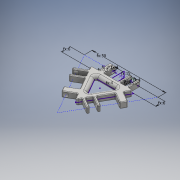
# Autodesk Inventor part: triangle
Saved by Autodesk Inventor 2016 (Build 200138000, 138)
## iProperties
Created: 2016-11-12
Part Number: triangle
Material: Generic
Document SubType Name: Modeling
Designer: Chris
Density: 1 g/cm^3
Appearance: Default
Author: Chris
Autodesk Inventor part; units mm, degrees
ref_plane "XZ Plane" through (0, 0, 0) normal (0, 1, 0) x (-1, 0, 0)
ref_plane "XY Plane" through (0, 0, 0) normal (0, 0, 1) x (1, 0, 0)
sketch "Sketch1" plane through (0, 0, 0) normal (0, 0, 1) x (1, 0, 0)
  line L0 (25, 14.4338) -> (0, -28.8675) construction
  line L1 (0, -28.8675) -> (-25, 14.4338) construction
  line L2 (-25, 14.4338) -> (25, 14.4338) construction
  line L3 (14.6077, 8.4338) -> (0, -16.8675)
  line L4 (0, -16.8675) -> (-14.6077, 8.4338)
  line L5 (-14.6077, 8.4338) -> (14.6077, 8.4338)
  line L6 (-7.5, 14.4338) -> (7.5, 14.4338) construction
  line L7 (5.5, 14.4338) -> (9.5, 14.4338) construction
  line L8 (-9.5, 14.4338) -> (-5.5, 14.4338) construction
  line L9 (7.6795, 4.4338) -> (0, -8.8675)
  line L10 (0, -8.8675) -> (-7.6795, 4.4338)
  line L11 (-7.6795, 4.4338) -> (7.6795, 4.4338)
  point P0 (0, 0)
  point P1 (0, 0)
  point P2 (0, 14.4338)
  dimension "d0" = 50
  dimension "d2" = 15
  dimension "d4" = 4
  dimension "d5" = 6
  dimension "d6" = 4
  dimension "d7" = 4
  dimension "d18" = 6
  constraints: 24 end point, 7 coincident, 4 horizontal, 4 midpoint, 1 collinear, 11 other
  measures "d0" distance of L1.end L0.start
  measures "d2" distance of L6.start L6.end
  measures "d4" distance of L7.start L7.end
  measures "d5" distance between parallel lines of L5 L7
  measures "d6" distance of L8.start L8.end
  measures "d7" distance between parallel lines of L5 L11
  measures "d18" distance between parallel lines of L5 L2
extrude "Extrusion1" add sketch "Sketch1" along normal mid plane 4
sketch "Sketch2" plane through (0, 0, 0) normal (1, 0, 0) x (0, 1, 0)
  line L0 (8.4338, 2) -> (8.4338, -2) construction
  line L1 (8.4338, -2) -> (8.4338, 2) construction
  line L2 (8.4338, 2) -> (13.4338, 2) construction
  line L3 (12.4338, -2) -> (8.4338, -2) construction
  line L4 (8.4338, -2) -> (8.4338, 2) construction
  arc A0 (14.4338, -2) -> (14.4338, 2) centre (14.4338, 0) ccw
  line L5 (14.4338, -2) -> (8.4338, -2)
  line L6 (8.4338, -2) -> (8.4338, 2)
  line L7 (8.4338, 2) -> (14.4338, 2)
  line L8 (14.4338, -2) -> (16.4338, -2)
  line L9 (16.4338, -2) -> (16.4338, 2)
  line L10 (16.4338, 2) -> (14.4338, 2)
  point P0 (0, 0)
  point P1 (14.4338, 0)
  point P2 (14.4338, 0)
  constraints: 18 end point, 5 perpendicular, 3 horizontal, 3 tangent, 2 coincident, 2 point on circle, 2 point on line, 1 centre point, 1 parallel
ref_plane "Work Plane1" through (-9.5, 14.4338, 0) normal (1, 0, 0) x (0, 1, 0)
ref_plane "Work Plane2" through (-5.5, 14.4338, 0) normal (1, 0, 0) x (0, 1, 0)
ref_plane "Work Plane3" through (5.5, 14.4338, 0) normal (1, 0, 0) x (0, 1, 0)
ref_plane "Work Plane4" through (9.5, 14.4338, 0) normal (1, 0, 0) x (0, 1, 0)
extrude "Extrusion2" add sketch "Sketch2" along normal up to surface (4 mm away) from surface at -9.5
ref_plane "Work Plane5" through (4, 14.4338, 0) normal (1, 0, 0) x (0, 1, 0)
ref_plane "Work Plane6" through (11, 14.4338, 0) normal (1, 0, 0) x (0, 1, 0)
extrude "Extrusion3" add sketch "Sketch2" along normal up to surface (1.5 mm away) from surface at 4
extrude "Extrusion4" add sketch "Sketch2" along normal up to surface (1.5 mm away) from surface at 9.5
sketch "Sketch3" plane through (0, 0, 0) normal (0, 0, 1) x (1, 0, 0)
  line L0 (-9.5, 15.9338) -> (-9.5, 14.4338)
  line L1 (-5.5, 15.9338) -> (-5.5, 14.4338)
  line L2 (5.5, 15.9338) -> (5.5, 14.4338)
  line L3 (9.5, 15.9338) -> (9.5, 14.4338)
  line L4 (5.5, 14.4338) -> (9.5, 14.4338) construction
  line L5 (-7.5, 14.4338) -> (7.5, 14.4338) construction
  arc A0 (6, 14.4338) -> (5.5, 15.9338) centre (3.5, 14.4338) ccw
  arc A1 (9.5, 15.9338) -> (9, 14.4338) centre (11.5, 14.4338) ccw
  arc A2 (-9, 14.4338) -> (-9.5, 15.9338) centre (-11.5, 14.4338) ccw
  arc A3 (-5.5, 15.9338) -> (-6, 14.4338) centre (-3.5, 14.4338) ccw
  line L6 (9, 14.4338) -> (9.5, 14.4338)
  line L7 (6, 14.4338) -> (5.5, 14.4338)
  line L8 (-5.5, 14.4338) -> (-6, 14.4338)
  line L9 (-9, 14.4338) -> (-9.5, 14.4338)
  point P0 (0, 0)
  point P1 (5.475, 16.4338)
  dimension "d31" = 0.5
  dimension "d32" = 3
  dimension "d33" = 0.5
  constraints: 16 end point, 8 point on circle, 5 collinear, 5 point on line, 4 centre point, 4 coincident, 4 vertical, 3 equal radius, 2 horizontal alignment
  measures "d31" distance of L2.end L7.start
  measures "d32" diameter of point (-9.5, 15.934) L9
  measures "d33" distance of L9.start L0.end
revolve "Revolution1" cut sketch "Sketch3" angle 360 about axis through (-9, 14.4338, 0) along (-1, 0, 0) contours A2 L9 L0 | L1 L8 A3
revolve "Revolution2" add sketch "Sketch3" angle 360 about axis through (6, 14.4338, 0) along (-1, 0, 0) contours A0 L7 L2 | L3 L6 A1
pattern_circular "Circular Pattern1" count 3 over 360 about axis through (0, 0, -10) along (0, 0, 1) of "Extrusion4", "Extrusion3", "Extrusion2", "Revolution1", "Revolution2"
fillet "Fillet2" radius 1 6 edges at (14.6077, 8.4338, 0) (-14.6077, 8.4338, 0) (0, -16.8675, 0) (7.6795, 4.4338, 0) (-7.6795, 4.4338, 0) (0, -8.8675, 0)
fillet "Fillet3" radius 0.5 36 edges at (2.5538, -12.4441, 0) (4.5538, -8.98, 0) (5.3038, -7.681, 0) (10.0538, 0.5463, 0) (12.0538, 4.0104, 0) (9.5, 8.4338, 0) (5.5, 8.4338, 0) (4, 8.4338, 0) (-5.5, 8.4338, 0) (-9.5, 8.4338, 0) (-12.0538, 4.0104, 0) (-10.0538, 0.5463, 0) (-9.3038, -0.7528, 0) (-4.5538, -8.98, 0) (-2.5538, -12.4441, 0) (-12.8038, 5.3094, 0) (11, 8.4338, 0) (1.8038, -13.7432, 0) (8.7321, -17.7432, 0) (9.4821, -16.4441, 0) (11.4821, -12.98, 0) (12.2321, -11.681, 0) (16.9821, -3.4537, 0) (18.9821, 0.0104, 0) (11, 16.4338, 0) (9.5, 16.4338, 0) (5.5, 16.4338, 0) (4, 16.4338, 0) (-5.5, 16.4338, 0) (-9.5, 16.4338, 0) (-19.7321, 1.3094, 0) (-18.9821, 0.0104, 0) (-16.9821, -3.4537, 0) (-16.2321, -4.7528, 0) (-11.4821, -12.98, 0) (-9.4821, -16.4441, 0)
fillet "Fillet4" radius 2 12 edges at (3.8397, -2.2169, -2) (0, -7.8675, -2) (-3.8397, -2.2169, -2) (-6.8135, 3.9338, -2) (0, 4.4338, -2) (6.8135, 3.9338, -2) (0, 4.4338, 2) (-6.8135, 3.9338, 2) (-3.8397, -2.2169, 2) (0, -7.8675, 2) (3.8397, -2.2169, 2) (6.8135, 3.9338, 2)
chamfer "Chamfer1" distance 0.4 angle 45 144 edges at (13.0227, 5.6885, 2) (13.7417, 7.9338, 2) (12.1878, 8.4338, 2) (11.1464, 8.5802, 2) (11, 12.4338, 2) (10.8536, 16.2873, 2) (9.6464, 16.2873, 2) (9.5, 12.4338, 2) (9.3536, 8.5802, 2) (7.5, 8.4338, 2) (5.6464, 8.5802, 2) (5.5, 12.4338, 2) (5.3536, 16.2873, 2) (4.1464, 16.2873, 2) (4, 12.4338, 2) (3.8536, 8.5802, 2) (-0.75, 8.4338, 2) (-5.3536, 8.5802, 2) (-5.5, 12.4338, 2) (-5.6464, 16.2873, 2) (-7.5, 16.4338, 2) (-9.3536, 16.2873, 2) (-9.5, 12.4338, 2) (-9.6464, 8.5802, 2) (-11.4378, 8.4338, 2) (-13.7417, 7.9338, 2) (-13.3977, 6.338, 2) (-13.0039, 5.363, 2) (-16.2679, 3.3094, 2) (-19.532, 1.2558, 2) (-18.9285, 0.2104, 2) (-15.5179, 2.0104, 2) (-12.1074, 3.8104, 2) (-11.0538, 2.2783, 2) (-10.2539, 0.5999, 2) (-13.5179, -1.4537, 2) (-16.782, -3.5073, 2) (-16.1785, -4.5528, 2) (-12.7679, -2.7528, 2) (-9.3574, -0.9528, 2) (-6.9288, -4.8664, 2) (-4.7539, -8.9264, 2) (-8.0179, -10.98, 2) (-11.282, -13.0336, 2) (-10.4821, -14.7121, 2) (-9.4285, -16.2441, 2) (-6.0179, -14.4441, 2) (-2.6074, -12.6441, 2) (-1.585, -14.1223, 2) (0, -15.8675, 2) (1.21, -14.7718, 2) (1.8574, -13.9432, 2) (5.2679, -15.7432, 2) (8.6785, -17.5431, 2) (9.282, -16.4977, 2) (6.0179, -14.4441, 2) (2.7539, -12.3905, 2) (3.5538, -10.7121, 2) (4.6074, -9.18, 2) (8.0179, -10.98, 2) (11.4285, -12.78, 2) (12.032, -11.7346, 2) (8.7679, -9.681, 2) (5.5039, -7.6274, 2) (7.6788, -3.5674, 2) (10.1074, 0.3463, 2) (13.5179, -1.4537, 2) (16.9285, -3.2537, 2) (17.9821, -1.7217, 2) (18.782, -0.0432, 2) (15.5179, 2.0104, 2) (12.2539, 4.064, 2) (13.5179, -1.4537, -2) (10.1074, 0.3463, -2) (7.6788, -3.5674, -2) (5.5039, -7.6274, -2) (8.7679, -9.681, -2) (12.032, -11.7346, -2) (11.4285, -12.78, -2) (8.0179, -10.98, -2) (4.6074, -9.18, -2) (3.5538, -10.7121, -2) (2.7539, -12.3905, -2) (6.0179, -14.4441, -2) (9.282, -16.4977, -2) (8.6785, -17.5431, -2) (5.2679, -15.7432, -2) (1.8574, -13.9432, -2) (1.21, -14.7718, -2) (0, -15.8675, -2) (-1.585, -14.1223, -2) (-2.6074, -12.6441, -2) (-6.0179, -14.4441, -2) (-9.4285, -16.2441, -2) (-10.4821, -14.7121, -2) (-11.282, -13.0336, -2) (-8.0179, -10.98, -2) (-4.7539, -8.9264, -2) (-6.9288, -4.8664, -2) (-9.3574, -0.9528, -2) (-12.7679, -2.7528, -2) (-16.1785, -4.5528, -2) (-16.782, -3.5073, -2) (-13.5179, -1.4537, -2) (-10.2539, 0.5999, -2) (-11.0538, 2.2783, -2) (-12.1074, 3.8104, -2) (-15.5179, 2.0104, -2) (-18.9285, 0.2104, -2) (-19.532, 1.2558, -2) (-16.2679, 3.3094, -2) (-13.0039, 5.363, -2) (-13.3977, 6.338, -2) (-13.7417, 7.9338, -2) (-11.4378, 8.4338, -2) (-9.6464, 8.5802, -2) (-9.5, 12.4338, -2) (-9.3536, 16.2873, -2) (-7.5, 16.4338, -2) (-5.6464, 16.2873, -2) (-5.5, 12.4338, -2) (-5.3536, 8.5802, -2) (-0.75, 8.4338, -2) (3.8536, 8.5802, -2) (4, 12.4338, -2) (4.1464, 16.2873, -2) (5.3536, 16.2873, -2) (5.5, 12.4338, -2) (5.6464, 8.5802, -2) (7.5, 8.4338, -2) (9.3536, 8.5802, -2) (9.5, 12.4338, -2) (9.6464, 16.2873, -2) (10.8536, 16.2873, -2) (11, 12.4338, -2) (11.1464, 8.5802, -2) (12.1878, 8.4338, -2) (13.7417, 7.9338, -2) (13.0227, 5.6885, -2) (12.2539, 4.064, -2) (15.5179, 2.0104, -2) (18.782, -0.0432, -2) (17.9821, -1.7217, -2) (16.9285, -3.2537, -2)
equation "\"d7\" = diam"
equation "\"d8\" = diam"
equation "\"d10\" = diam"
equation "\"d14\" = diam"
equation "\"d16\" = diam"
equation "\"diam\" = 4"
equation "\"dent\" = 0.5"
equation "\"matespace\" = 15"
equation "\"springwidth\" = 1.5"
equation "\"fingerwidth\" = 4"
equation "\"tolerance\" = 0"
equation "\"dentdiam\" = 3"
equation "\"springlength\" = 6"
body "Solid1"
